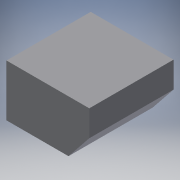
# Autodesk Inventor part: Case 2
Saved by Autodesk Inventor 2017 (Build 210142000, 142)
## iProperties
Created: 2017-04-30
Part Number: Case 2
Material: Generic
Document SubType Name: Modeling
Designer: X220T
Density: 1 g/cm^3
Appearance: Default
Author: X220T
Autodesk Inventor part; units mm, degrees
ref_plane "YZ Plane" through (0, 0, 0) normal (1, 0, 0) x (0, 1, 0)
ref_plane "XZ Plane" through (0, 0, 0) normal (0, 1, 0) x (-1, 0, 0)
ref_plane "XY Plane" through (0, 0, 0) normal (0, 0, 1) x (1, 0, 0)
sketch "Sketch1" plane through (0, 0, 0) normal (0, 1, 0) x (-1, 0, 0)
  line L0 (0, 0) -> (53.5, 0)
  line L1 (53.5, 0) -> (53.5, 44)
  line L2 (53.5, 44) -> (-19.5, 44)
  line L3 (-19.5, 44) -> (-19.5, 21)
  line L4 (-19.5, 21) -> (0, 0)
  dimension "d3" = 53.5
  dimension "d4" = 44
  dimension "d5" = 23
  dimension "d6" = 73
  constraints: 10 end point, 3 perpendicular, 1 horizontal
  measures "d3" distance of L0.start L0.end
  measures "d4" distance of L0.end L1.end
  measures "d5" distance of L2.end L3.end
  measures "d6" distance of L1.end L2.end
extrude "Extrusion1" add sketch "Sketch1" along normal mid plane 55
draft "FaceDraft1" angle 20 pull direction (0, 0, -1) faces at (-11.3333, 27.5, 29.3333) (-11.3333, -27.5, 29.3333) fixed edges at (-26.75, 27.5, 0) (-26.75, -27.5, 0)
sketch "Sketch2" plane through (-53.5, 43.5147, 44) normal (0, 0, 1) x (1, 0, 0)
  circle A0 centre (44.2818, -14.0647) radius 1.5 projected
  circle A1 centre (10.2818, -14.0647) radius 1.5 projected
  circle A2 centre (10.2818, -72.9647) radius 1.5 projected
  circle A3 centre (44.2818, -72.9647) radius 1.5 projected
  point P0 (53.5, -43.5147)
extrude "Extrusion2" cut sketch "Sketch2" against normal blind 10.11
sketch "Sketch3" plane through (-53.5, 43.5147, 44) normal (0, 0, 1) x (1, 0, 0)
  circle A0 centre (44.2818, -14.0647) radius 1.5 projected
  circle A1 centre (44.2818, -14.0647) radius 3.25
  circle A2 centre (10.2818, -14.0647) radius 1.5 projected
  circle A3 centre (10.2818, -14.0647) radius 3.25
  circle A4 centre (10.2818, -72.9647) radius 1.5 projected
  circle A5 centre (10.2818, -72.9647) radius 3.25
  circle A6 centre (44.2818, -72.9647) radius 1.5 projected
  circle A7 centre (44.2818, -72.9647) radius 3.25
  point P0 (53.5, -43.5147)
  dimension "d10" = 6.5
  constraints: 4 centre point, 4 coincident, 3 equal radius
  measures "d10" diameter of A1
extrude "Extrusion3" cut sketch "Sketch3" against normal blind 9
shell "Shell1" thickness 1.5 removed faces 5 at (19.5, -11.7145, 36.3333) at (13, 9.1667, 14) at (-35.6667, 32.8382, 14.6667) at (-35.6667, -32.8382, 14.6667) at (-17.8333, -9.1667, 0)
chamfer "Chamfer1" distance 3 angle 45 4 edges at (-13.9682, -29.45, 42.5) (-47.9682, -29.45, 42.5) (-13.9682, 29.45, 42.5) (-47.9682, 29.45, 42.5)
chamfer "Chamfer2" distance 1 angle 45 4 edges at (-12.2182, -29.45, 33.5) (-46.2182, -29.45, 33.5) (-12.2182, 29.45, 33.5) (-46.2182, 29.45, 33.5)
sketch "Sketch4" plane through (-9.2182, -29.45, 33.89) normal (0, 0, 1) x (1, 0, 0)
  circle A0 centre (0, 0) radius 1.5 construction
  circle A1 centre (-34, 0) radius 1.5 construction
  circle A2 centre (0, 58.9) radius 1.5 construction
  circle A3 centre (-34, 58.9) radius 1.5 construction
  circle A4 centre (-34, 58.9) radius 1.75
  circle A5 centre (0, 58.9) radius 1.75
  circle A6 centre (0, 0) radius 1.75
  circle A7 centre (-34, 0) radius 1.75
  point P0 (9.2182, 29.45)
  dimension "d19" = 3.5
  constraints: 4 centre point, 3 equal radius
  measures "d19" diameter of A4
extrude "Extrusion4" cut sketch "Sketch4" along normal through all both and the other way through all
chamfer "Chamfer3" distance 3 angle 45 1 edges at (-52, 0, 42.5)
sketch "Sketch5" plane through (-53.5, -43.5147, 44) normal (-1, 0, 0) x (0, 0, 1)
  line L0 (-33.6389, 49.1201) -> (-11.6389, 49.1201)
  line L1 (-11.6389, 49.1201) -> (-11.6389, 46.3701)
  line L2 (-11.6389, 46.3701) -> (-33.6389, 46.3701)
  line L3 (-33.6389, 46.3701) -> (-33.6389, 49.1201)
  point P0 (-44, 43.5147)
  dimension "d25" = 22
  dimension "d26" = 2.75
  constraints: 8 end point, 2 parallel, 1 horizontal, 1 perpendicular
  measures "d25" distance of L1.end L2.end
  measures "d26" distance of L0.end L1.end
extrude "Extrusion5" cut sketch "Sketch5" against normal blind 9
body "Solid1"
